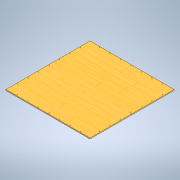
# Autodesk Inventor part: Bottom_Plate
Saved by Autodesk Inventor 2021.3 (Build 253353000, 353)
## iProperties
Created: 2022-01-11
Part Number: Bottom_Plate
Material: Bamboo
Document SubType Name: Modeling
Designer: nxf77172
Density: 0.7 g/cm^3
Appearance: Bamboo
Author: nxf77172
Autodesk Inventor part; units mm, degrees
ref_plane "YZ Plane" through (0, 0, 0) normal (1, 0, 0) x (0, 1, 0)
ref_plane "XZ Plane" through (0, 0, 0) normal (0, 1, 0) x (-1, 0, 0)
ref_plane "XY Plane" through (0, 0, 0) normal (0, 0, 1) x (1, 0, 0)
sketch "Sketch1" plane through (0, 0, 0) normal (0, 1, 0) x (-1, 0, 0)
  line L0 (350, 350) -> (-350, 350)
  line L1 (-350, 350) -> (-350, -350)
  line L2 (-350, -350) -> (350, -350)
  line L3 (350, -350) -> (350, 350)
  line L4 (350, 350) -> (-350, -350) construction
  line L5 (-350, 350) -> (350, -350) construction
  line L6 (-329, 350) -> (-329, 329)
  line L7 (-329, 329) -> (-350, 329)
  line L8 (-350, -329) -> (-329, -329)
  line L9 (-329, -329) -> (-329, -350)
  line L10 (329, -350) -> (329, -329)
  line L11 (329, -329) -> (350, -329)
  line L12 (350, 329) -> (329, 329)
  line L13 (329, 329) -> (329, 350)
  line L14 (-350, 251) -> (-329, 251)
  line L15 (-329, 251) -> (-329, 251)
  line L16 (-329, 209) -> (-350, 209)
  line L17 (-329, 209) -> (-329, 251)
  line L18 (350, 0) -> (-350, 0) construction
  line L19 (0, -350) -> (0, 350) construction
  line L20 (-350, -251) -> (-329, -251)
  line L21 (-329, -209) -> (-350, -209)
  line L22 (-329, -209) -> (-329, -251)
  line L23 (0, 350) -> (0, -350) construction
  line L24 (350, 251) -> (329, 251)
  line L25 (329, 251) -> (329, 251)
  line L26 (329, 209) -> (350, 209)
  line L27 (329, 209) -> (329, 251)
  line L28 (329, -209) -> (350, -209)
  line L29 (329, -209) -> (329, -251)
  line L30 (350, -251) -> (329, -251)
  line L31 (-350, 340) -> (350, 340) construction
  circle A0 centre (262.5, 340) radius 2
  circle A1 centre (175, 340) radius 2
  circle A2 centre (87.5, 340) radius 2
  circle A3 centre (0, 340) radius 2
  circle A4 centre (-262.5, 340) radius 2
  circle A5 centre (-175, 340) radius 2
  circle A6 centre (-87.5, 340) radius 2
  line L32 (-340, -350) -> (-340, 350) construction
  circle A7 centre (-340, -175) radius 2
  circle A8 centre (-340, 0) radius 2
  circle A9 centre (-340, 87.5) radius 2
  circle A10 centre (-340, -87.5) radius 2
  circle A11 centre (-340, -262.5) radius 2
  circle A12 centre (-340, 175) radius 2
  circle A13 centre (-340, 262.5) radius 2
  line L33 (350, -340) -> (-350, -340) construction
  circle A14 centre (175, -340) radius 2
  circle A15 centre (0, -340) radius 2
  circle A16 centre (-87.5, -340) radius 2
  circle A17 centre (87.5, -340) radius 2
  circle A18 centre (262.5, -340) radius 2
  circle A19 centre (-175, -340) radius 2
  circle A20 centre (-262.5, -340) radius 2
  line L34 (340, 350) -> (340, -350) construction
  circle A21 centre (340, 175) radius 2
  circle A22 centre (340, 0) radius 2
  circle A23 centre (340, -87.5) radius 2
  circle A24 centre (340, 87.5) radius 2
  circle A25 centre (340, 262.5) radius 2
  circle A26 centre (340, -175) radius 2
  circle A27 centre (340, -262.5) radius 2
  line L35 (350, 220) -> (-350, 220) construction
  line L36 (350, 280) -> (-350, 280) construction
  circle A28 centre (262.5, 220) radius 2
  circle A29 centre (175, 220) radius 2
  circle A30 centre (87.5, 220) radius 2
  circle A31 centre (0, 220) radius 2
  circle A32 centre (-262.5, 220) radius 2
  circle A33 centre (-175, 220) radius 2
  circle A34 centre (-87.5, 220) radius 2
  circle A35 centre (175, -220) radius 2
  circle A36 centre (262.5, -220) radius 2
  circle A37 centre (-262.5, -220) radius 2
  circle A38 centre (-175, -220) radius 2
  circle A39 centre (87.5, -220) radius 2
  circle A40 centre (-87.5, -220) radius 2
  circle A41 centre (0, -220) radius 2
  line L37 (12.5, 160) -> (-12.5, 160)
  line L38 (-12.5, 160) -> (-12.5, 210)
  line L39 (-12.5, 210) -> (12.5, 210)
  line L40 (12.5, 210) -> (12.5, 160)
  line L41 (12.5, 160) -> (-12.5, 210) construction
  line L42 (-12.5, 160) -> (12.5, 210) construction
  line L43 (12.5, -160) -> (-12.5, -160)
  line L44 (-12.5, -160) -> (-12.5, -210)
  line L45 (-12.5, -210) -> (12.5, -210)
  line L46 (12.5, -210) -> (12.5, -160)
  point P0 (0, 0)
  point P1 (0, 0)
  point P2 (-350, -209)
  point P3 (350, -209)
  point P4 (350, 209)
  point P5 (0, 185)
  dimension "d0" = 700
  dimension "d1" = 700
  dimension "d2" = 21
  dimension "d3" = 21
  dimension "d6" = 360
  dimension "d8" = 21
  dimension "d9" = 99
  dimension "d10" = 141
  dimension "d13" = 10
  dimension "d14" = 4
  dimension "d15" = 4
  dimension "d16" = 4
  dimension "d17" = 175
  dimension "d18" = 87.5
  dimension "d19" = 87.5
  dimension "d20" = 4
  dimension "d23" = 360
  dimension "d25" = 130
  dimension "d26" = 120
  dimension "d27" = 60
  dimension "d28" = 140
  dimension "d29" = 25
  dimension "d30" = 50
  constraints: 92 end point, 42 centre point, 35 symmetric about line, 17 point on line, 7 horizontal, 7 midpoint, 4 perpendicular, 3 parallel, 2 vertical, 1 coincident, 117 other
  measures "d0" distance of L0.start L0.end
  measures "d1" distance of L2.end L0.start
  measures "d2" distance of L6.start L6.end
  measures "d3" distance of L6.end L7.end
  measures "d8" distance of L14.start L14.end
  measures "d9" distance between parallel lines of L0 L14
  measures "d10" distance between parallel lines of L0 L16
  measures "d13" distance between parallel lines of L31 L0
  measures "d14" diameter of A0
  measures "d15" diameter of A1
  measures "d16" diameter of A2
  measures "d17" distance from line of L19 A1.centre
  measures "d18" distance from line of A2.centre L19
  measures "d19" distance from line of A0.centre L3
  measures "d20" diameter of A3
  measures "d25" distance between parallel lines of L0 L35
  measures "d26" distance between parallel lines of L35 L31
  measures "d27" distance between parallel lines of L35 L36
  measures "d28" distance between parallel lines of L39 L0
  measures "d29" distance between parallel lines of L38 L40
  measures "d30" distance between parallel lines of L39 L37
extrude "Extrusion1" add sketch "Sketch1" along normal blind 8 contours L3 L12 L13 L0 | L13 L12 L3 L24 L27 L26 L28 L29 L30 L11 L10 L2 L9 L8 L1 L20 L22 L21 L16 L17 L14 L7 L6 L0 | L6 L7 L1 L0 | L3 L26 L27 L24 | L3 L30 L29 L28 | L14 L17 L16 L1 | L3 L2 L10 L11 | L21 L22 L20 L1 | L8 L9 L2 L1 | A28 | A29 | A30 | A31 | A32 | A33 | A34 | A35 | A36 | A37 | A38 | A39 | A40 | A41 | L37 L38 L39 L40 | L46 L45 L44 L43
equation "\"d1\" = d0"
equation "\"d3\" = d2"
equation "\"d15\" = d14"
equation "\"d16\" = d14"
equation "\"d18\" = 0.5 * d17"
equation "\"d19\" = d18"
equation "\"d20\" = d14"
equation "\"d27\" = 0.5 * d26"
body "Solid1"
